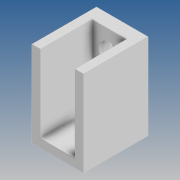
# Autodesk Inventor part: WaterDrainWellMount
Saved by Autodesk Inventor 2020 (Build 240168000, 168)
## iProperties
Created: 2019-08-08
Part Number: WaterDrainWellMount
Material: 일반
Document SubType Name: Modeling
Designer: Jeong Ji Hoon
Density: 1 g/cm^3
Appearance: 기본값
Author: Jeong Ji Hoon
## iProperties of the stored document _3D 인쇄.ipt
Created: 2019-08-08
Part Number: _3D 인쇄
Material: 일반
Document SubType Name: Modeling
Designer: Jeong Ji Hoon
Density: 1 g/cm^3
Appearance: 기본값
Author: Jeong Ji Hoon
Autodesk Inventor part; units mm, degrees
ref_plane "YZ Plane" through (0, 0, 0) normal (1, 0, 0) x (0, 1, 0)
ref_plane "XZ Plane" through (0, 0, 0) normal (0, 1, 0) x (-1, 0, 0)
ref_plane "XY Plane" through (0, 0, 0) normal (0, 0, 1) x (1, 0, 0)
sketch "스케치1" plane through (0, 0, 0) normal (0, 0, 1) x (1, 0, 0)
  line L0 (0, 0) -> (12, 0)
  line L1 (12, 0) -> (12, 20)
  line L2 (12, 20) -> (0, 20)
  line L3 (0, 20) -> (0, 0)
  dimension "d0" = 12
  dimension "d1" = 20
  constraints: 8 end point, 2 parallel, 1 horizontal, 1 perpendicular
  measures "d0" distance of L2.end L1.end
  measures "d1" distance of L1.end L0.end
extrude "돌출1" add sketch "스케치1" along normal blind 3
sketch "스케치2" plane through (0, 0, 3) normal (0, 0, 1) x (1, 0, 0)
  line L0 (0, 20) -> (0, 0) projected
  line L1 (0, 0) -> (12, 0) projected
  line L2 (12, 0) -> (12, 20) projected
  line L3 (12, 20) -> (0, 20) projected
  line L4 (2, 20) -> (2, 0)
  line L5 (10, 20) -> (10, 0)
  line L6 (2, 2) -> (10, 2)
  dimension "d4" = 2
  dimension "d5" = 2
  dimension "d6" = 2
  constraints: 6 end point, 6 point on line, 3 perpendicular
  measures "d4" distance between parallel lines of L0 L4
  measures "d5" distance between parallel lines of L2 L5
  measures "d6" distance between parallel lines of L1 L6
extrude "돌출2" add sketch "스케치2" along normal blind 12 contours L3 L4 L1 L0 | L4 L6 L5 L1 | L3 L2 L1 L5
sketch "스케치3" plane through (0, 0, 0) normal (0, 0, -1) x (-1, 0, 0)
  line L0 (0, 0) -> (-12, 0) projected
  circle A0 centre (-6, 5) radius 2.45
  circle A1 centre (-6, 15) radius 2.45
  point P0 (-6, 0)
  point P1 (-6, 0)
  dimension "d9" = 5
  dimension "d10" = 10
  dimension "d11" = 4.9
  dimension "d12" = 4.9
  constraints: 2 centre point, 2 midpoint, 2 vertical alignment
  measures "d9" distance from line of L0 A0.centre
  measures "d10" distance of A1.centre A0.centre
  measures "d11" diameter of A0
  measures "d12" diameter of A1
extrude "돌출3" cut sketch "스케치3" against normal blind 3
